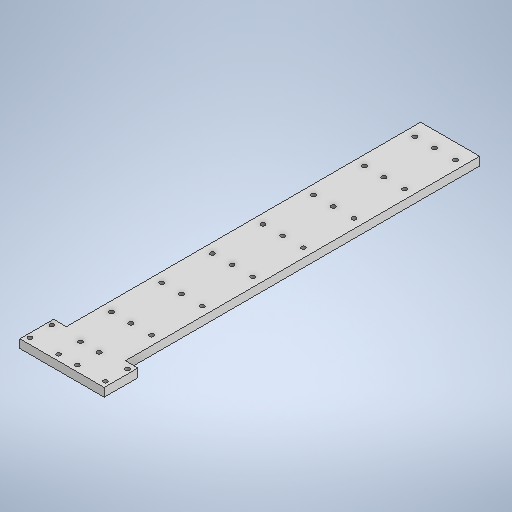
# Autodesk Inventor part: plaskownik_uchwyt_silownika_L460_W100_H10
Saved by Autodesk Inventor 2025.2 (Build 292293000, 293)
## iProperties
Created: 2025-03-20
Part Number: plaskownik_uchwyt_silownika_L460_W100_H10
Material: Ogólny
Document SubType Name: Modeling
Designer: rango
Density: 1 g/cm^3
Appearance: Domyślna
Author: rango
Autodesk Inventor part; units mm, degrees
ref_plane "YZ Plane" through (0, 0, 0) normal (1, 0, 0) x (0, 1, 0)
ref_plane "XZ Plane" through (0, 0, 0) normal (0, 1, 0) x (-1, 0, 0)
ref_plane "XY Plane" through (0, 0, 0) normal (0, 0, 1) x (1, 0, 0)
sketch "Szkic3" plane through (0, 0, 0) normal (0, 1, 0) x (-1, 0, 0)
  line L0 (50, 20) -> (-50, 20)
  line L1 (-50, 20) -> (-50, -20)
  line L2 (-50, -20) -> (50, -20)
  line L3 (50, -20) -> (50, 20)
  point P0 (0, 0)
  dimension "d4" = 100
  dimension "d5" = 40
  constraints: 8 end point, 2 parallel, 1 horizontal, 1 perpendicular
  measures "d4" distance of L2.end L1.end
  measures "d5" distance of L1.end L0.end
extrude "Wyciągnięcie proste1" add sketch "Szkic3" along normal blind 10
sketch "Szkic4" plane through (0, 10, 0) normal (0, 1, 0) x (1, 0, 0)
  line L0 (50, 20) -> (-50, 20) projected
  line L1 (35.1646, 20) -> (-34.8354, 20)
  line L2 (-34.8354, 20) -> (-34.8354, 440)
  line L3 (-34.8354, 440) -> (35.1646, 440)
  line L4 (35.1646, 440) -> (35.1646, 20)
  point P0 (0, 0)
  dimension "d8" = 70
  dimension "d9" = 420
  constraints: 8 end point, 2 parallel, 1 horizontal, 1 perpendicular, 1 point on line
  measures "d8" distance of L2.end L3.end
  measures "d9" distance of L1.end L2.end
extrude "Wyciągnięcie proste2" add sketch "Szkic4" against normal blind 10
sketch "Szkic5" plane through (0, 10, 0) normal (0, 1, 0) x (1, 0, 0)
  line L0 (0, 13) -> (0, -13) construction
  circle A0 centre (-45, 13) radius 2.5
  circle A1 centre (-45, -13) radius 2.5
  circle A2 centre (45, 13) radius 2.5
  circle A3 centre (44.4361, -13) radius 2.5
  line L1 (-45, 13) -> (-11, 13) construction
  line L2 (45, 13) -> (11, 13) construction
  circle A4 centre (-11, 13) radius 2.5
  circle A5 centre (-11, -13) radius 2.5
  circle A6 centre (11, -13) radius 2.5
  circle A7 centre (11, 13) radius 2.5
  point P0 (0, 0)
  dimension "d12" = 26
  dimension "d13" = 5
  dimension "d14" = 5
  dimension "d15" = 5
  dimension "d16" = 5
  dimension "d17" = 34
  dimension "d18" = 34
  dimension "d19" = 5
  dimension "d20" = 5
  dimension "d21" = 5
  dimension "d22" = 5
  constraints: 8 centre point, 6 end point, 2 coincident, 2 horizontal, 1 vertical
  measures "d12" distance of L0.start L0.end
  measures "d13" diameter of A0
  measures "d14" diameter of A1
  measures "d15" diameter of A2
  measures "d16" diameter of A3
  measures "d17" distance of L1.start L1.end
  measures "d18" distance of L2.start L2.end
  measures "d19" diameter of A4
  measures "d20" diameter of A5
  measures "d21" diameter of A6
  measures "d22" diameter of A7
hole "Otwór1" at (-45, 10, -13) at (-45, 10, 13) at (-11, 10, 13) at (-11, 10, -13) at (11, 10, -13) at (11, 10, 13) at (44.4361, 10, 13) at (45, 10, -13) direction (0, -1, 0) diameter 4.9784 depth 10 tip angle 118 thread size "1/4-20 UNC" class "2B" standard "ANSI Unified Screw Threads"
sketch "Szkic6" plane through (0, 10, 0) normal (0, 1, 0) x (1, 0, 0)
  line L0 (35.1646, 440) -> (35.1646, 20) projected
  line L1 (35.1646, 61.6763) -> (-34.8354, 61.6763) construction
  line L2 (-34.8354, 20) -> (-34.8354, 440) projected
  line L3 (24.5428, 61.6763) -> (-23.3042, 61.6763) construction
  circle A0 centre (-23.3042, 61.6763) radius 4
  circle A1 centre (24.5428, 61.6763) radius 4
  circle A2 centre (-23.3042, 121.6763) radius 4
  circle A3 centre (24.5428, 121.6763) radius 4
  circle A4 centre (-23.3042, 181.6763) radius 4
  circle A5 centre (24.5428, 181.6763) radius 4
  circle A6 centre (-23.3042, 241.6763) radius 4
  circle A7 centre (24.5428, 241.6763) radius 4
  circle A8 centre (-23.3042, 301.6763) radius 4
  circle A9 centre (24.5428, 301.6763) radius 4
  circle A10 centre (-23.3042, 361.6763) radius 4
  circle A11 centre (24.5428, 361.6763) radius 4
  circle A12 centre (-23.3042, 421.6763) radius 4
  circle A13 centre (24.5428, 421.6763) radius 4
  circle A14 centre (0, 61.6763) radius 4
  circle A15 centre (0, 121.6763) radius 4
  circle A16 centre (0, 181.6763) radius 4
  circle A17 centre (0, 241.6763) radius 4
  circle A18 centre (0, 301.6763) radius 4
  circle A19 centre (0, 361.6763) radius 4
  circle A20 centre (0, 421.6763) radius 4
  point P0 (0, 0)
  point P1 (-27.7985, 121.5078)
  point P2 (8.1646, 122)
  point P3 (-27.8354, 182)
  point P4 (8.1646, 182)
  point P5 (-27.8354, 242)
  point P6 (8.1646, 242)
  point P7 (-27.8354, 302)
  point P8 (8.1646, 302)
  point P9 (-27.8354, 362)
  point P10 (8.1646, 362)
  point P11 (-27.8354, 422)
  point P12 (8.1646, 422)
  dimension "d30" = 47.847
  dimension "d45" = 8
  dimension "d49" = 60
  dimension "d61" = 8
  dimension "d64" = 60
  dimension "d76" = 8
  dimension "d79" = 60
  constraints: 21 centre point, 5 point on line, 4 end point, 2 coincident, 2 vertical, 1 horizontal, 36 other
  measures "d30" distance of L3.start L3.end
  measures "d45" diameter of A0
  measures "d49" distance of A0.centre point (-27.798, 121.508)
  measures "d61" diameter of A1
  measures "d64" distance of A0.centre A2.centre
  measures "d76" diameter of A14
  measures "d79" distance of A14.centre A15.centre
hole "Otwór5" at (-23.3042, 10, -61.6763) at (0, 10, -61.6763) at (24.5428, 10, -61.6763) at (-23.3042, 10, -121.6763) at (0, 10, -121.6763) at (24.5428, 10, -121.6763) at (-23.3042, 10, -181.6763) at (0, 10, -181.6763) at (24.5428, 10, -181.6763) at (-23.3042, 10, -241.6763) at (0, 10, -241.6763) at (24.5428, 10, -241.6763) at (-23.3042, 10, -301.6763) at (0, 10, -301.6763) at (24.5428, 10, -301.6763) at (-23.3042, 10, -361.6763) at (0, 10, -361.6763) at (24.5428, 10, -361.6763) at (-23.3042, 10, -421.6763) at (0, 10, -421.6763) at (24.5428, 10, -421.6763) direction (0, -1, 0) diameter 4.9784 depth 50 tip angle 118 thread size "1/4-20 UNC" class "2B" standard "ANSI Unified Screw Threads"
